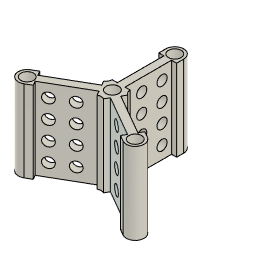
CanSat_MK.2 v2 v7 (Autodesk Fusion 360 archive; units mm, degrees)
design "Module"
Autodesk Fusion 360 part; units mm, degrees
sketch "Sketch1" plane through (0, 0, 0) normal (0, 0, 1) x (1, 0, 0)
  circle A0 centre (0, 0) radius 32
  circle A1 centre (0, 24.5) radius 2.5
  circle A2 centre (-21.2176, -12.25) radius 2.5
  circle A3 centre (21.2176, -12.25) radius 2.5
  circle A4 centre (0, 0) radius 2.5
  line L0 (-3.5, 3.4641) -> (-3.5, 24.5)
  line L1 (3.5, 24.5) -> (3.5, 3.4641)
  line L2 (-1.25, -4.7631) -> (-19.4676, -15.2811)
  line L3 (-22.9676, -9.2189) -> (-4.75, 1.299)
  line L4 (4.75, 1.299) -> (22.9676, -9.2189)
  line L5 (19.4676, -15.2811) -> (1.25, -4.7631)
  arc A5 (-4.75, 1.299) -> (-3.5, 3.4641) centre (-6, 3.4641) ccw
  arc A6 (3.5, 3.4641) -> (4.75, 1.299) centre (6, 3.4641) ccw
  arc A7 (1.25, -4.7631) -> (-1.25, -4.7631) centre (0, -6.9282) ccw
  arc A8 (3.5, 24.5) -> (-3.5, 24.5) centre (0, 24.5) ccw
  arc A9 (19.4676, -15.2811) -> (22.9676, -9.2189) centre (21.2176, -12.25) ccw
  arc A10 (-22.9676, -9.2189) -> (-19.4676, -15.2811) centre (-21.2176, -12.25) ccw
  dimension "d1" = 64
  dimension "d2" = 24.5
  dimension "d3" = 5
  dimension "d5" = 360
  dimension "d6" = 7
  dimension "d8" = 360
  dimension "d10" = 5
  dimension "d15" = 2.5
  dimension "d16" = 2.5
  dimension "d17" = 2.5
  constraint coincident A0.centre A4.centre
  constraint concentric A1 A8
  constraint vertical L0
  constraint vertical L1
  constraint tangent L0 A5
  constraint tangent L3 A5
  constraint tangent L1 A6
  constraint tangent L4 A6
  constraint tangent L5 A7
  constraint tangent L2 A7
  measures "d1" diameter of A0
  measures "d2" distance of A0.centre A1.centre
  measures "d3" diameter of A1
  measures "d6" diameter of A8
  measures "d10" diameter of A4
  measures "d15" radius of A5
  measures "d16" radius of A6
  measures "d17" radius of A7
extrude "Extrude1" add sketch "Sketch1" along normal blind 32 contours L0 L1 L2 L3 L4 L5 A5 A6 A7 A8 A9 A10
sketch "Sketch2" plane through (1.75, -3.0311, 0) normal (0.5, -0.866025, 0) x (0.866025, 0.5, 0)
  line L0 (-24.5, 0) -> (-3.4641, 0)
  line L1 (-3.4641, 0) -> (-3.4641, 32)
  line L2 (-3.4641, 32) -> (-24.5, 32)
  line L3 (-24.5, 32) -> (-24.5, 0)
  line L4 (-24.5, 32) -> (-3.4641, 32)
  line L5 (-3.4641, 32) -> (-3.4641, 0)
  line L6 (-3.4641, 0) -> (-24.5, 0)
  line L7 (-24.5, 0) -> (-24.5, 32)
  circle A0 centre (-18, 27) radius 2
  circle A1 centre (-10, 27) radius 2
  circle A2 centre (-18, 19.6667) radius 2
  circle A3 centre (-10, 19.6667) radius 2
  circle A4 centre (-18, 12.3333) radius 2
  circle A5 centre (-10, 12.3333) radius 2
  circle A6 centre (-18, 5) radius 2
  circle A7 centre (-10, 5) radius 2
  dimension "d20" = 4
  dimension "d23" = 8
  dimension "d24" = -22
  constraint horizontal L4
  constraint vertical L5
  constraint horizontal L6
  constraint vertical L7
  constraint coincident L0.end L1.start
  constraint coincident L2.end L3.start
  measures "d20" diameter of A0
extrude "Extrude2" cut sketch "Sketch2" against normal blind 8 contours A0 | A1 | A2 | A3 | A4 | A5 | A6 | A7
pattern_circular "C-Pattern1" count 3 over 360 about axis through (0, 0, 1.75) along (0, 0, 1) of "Extrude2"
sketch "Sketch3" plane through (1.75, -3.0311, 0) normal (0.5, -0.866025, 0) x (0.866025, 0.5, 0)
  circle A0 centre (-10, 12.3333) radius 2
  circle A1 centre (-10, 27) radius 2
  circle A2 centre (-18, 19.6667) radius 2
  circle A3 centre (-10, 5) radius 2
  circle A4 centre (-18, 12.3333) radius 2
  circle A5 centre (-18, 27) radius 2
  circle A6 centre (-10, 19.6667) radius 2
  circle A7 centre (-18, 5) radius 2
  line L0 (-24.5, 0) -> (-3.4641, 0)
  line L1 (-3.4641, 0) -> (-3.4641, 32)
  line L2 (-3.4641, 32) -> (-24.5, 32)
  line L3 (-24.5, 32) -> (-24.5, 0)
  line L4 (-21.8286, 32) -> (-21.8286, 0)
  constraint coincident L2 L4.start
  constraint coincident L0 L4.end
  constraint perpendicular L0 L4
extrude "Extrude3" cut sketch "Sketch3" against normal blind 2 contours L0 L1 L2 L4
sketch "Sketch5" plane through (-1.75, 3.0311, 0) normal (-0.5, 0.866025, 0) x (-0.866025, -0.5, 0)
  circle A0 centre (10, 12.3333) radius 2
  circle A1 centre (10, 27) radius 2
  circle A2 centre (18, 19.6667) radius 2
  circle A3 centre (10, 5) radius 2
  circle A4 centre (18, 12.3333) radius 2
  circle A5 centre (18, 27) radius 2
  circle A6 centre (10, 19.6667) radius 2
  circle A7 centre (18, 5) radius 2
  line L0 (3.4641, 0) -> (24.5, 0)
  line L1 (24.5, 0) -> (24.5, 32)
  line L2 (24.5, 32) -> (3.4641, 32)
  line L3 (3.4641, 32) -> (3.4641, 0)
  line L4 (24.5, 32) -> (21.829, 32)
  line L5 (21.829, 32) -> (21.829, 0)
  dimension "d31" = 2.671
  constraint coincident L1.end L2.start
  constraint perpendicular L1 L4
  constraint coincident L0 L5.end
  constraint perpendicular L0 L5
  measures "d31" distance of L1.end L4.end
extrude "Extrude4" cut sketch "Sketch5" against normal blind 2 contours L0 L2 L3 L5
sketch "Sketch6" plane through (-3.5, 0, 0) normal (-1, 0, 0) x (0, -1, 0)
  circle A0 centre (-10, 12.3333) radius 2
  circle A1 centre (-10, 27) radius 2
  circle A2 centre (-18, 19.6667) radius 2
  circle A3 centre (-10, 5) radius 2
  circle A4 centre (-18, 12.3333) radius 2
  circle A5 centre (-18, 27) radius 2
  circle A6 centre (-10, 19.6667) radius 2
  circle A7 centre (-18, 5) radius 2
  line L0 (-24.5, 0) -> (-3.4641, 0)
  line L1 (-3.4641, 0) -> (-3.4641, 32)
  line L2 (-3.4641, 32) -> (-24.5, 32)
  line L3 (-24.5, 32) -> (-24.5, 0)
  line L4 (-24.5, 32) -> (-21.739, 32)
  line L5 (-21.739, 32) -> (-21.739, 0)
  dimension "d34" = 2.761
  constraint coincident L2.end L3.start
  constraint perpendicular L3 L4
  constraint coincident L0 L5.end
  constraint perpendicular L0 L5
  measures "d34" distance of L2.end L4.end
extrude "Extrude5" cut sketch "Sketch6" against normal blind 2 contours L0 L1 L2 L5
sketch "Sketch7" plane through (3.5, 0, 0) normal (1, 0, 0) x (0, 1, 0)
  circle A0 centre (10, 12.3333) radius 2
  circle A1 centre (10, 27) radius 2
  circle A2 centre (18, 19.6667) radius 2
  circle A3 centre (10, 5) radius 2
  circle A4 centre (18, 12.3333) radius 2
  circle A5 centre (18, 27) radius 2
  circle A6 centre (10, 19.6667) radius 2
  circle A7 centre (18, 5) radius 2
  line L0 (3.4641, 0) -> (24.5, 0)
  line L1 (24.5, 0) -> (24.5, 32)
  line L2 (24.5, 32) -> (3.4641, 32)
  line L3 (3.4641, 32) -> (3.4641, 0)
  line L4 (24.5, 32) -> (21.739, 32)
  line L5 (21.739, 32) -> (21.739, 0)
  dimension "d37" = 2.761
  constraint coincident L1.end L2.start
  constraint perpendicular L1 L4
  constraint coincident L0 L5.end
  constraint perpendicular L0 L5
  measures "d37" distance of L1.end L4.end
extrude "Extrude6" cut sketch "Sketch7" against normal blind 2 contours L0 L2 L3 L5
sketch "Sketch8" plane through (1.75, 3.0311, 0) normal (0.5, 0.866025, 0) x (-0.866025, 0.5, 0)
  circle A0 centre (-10, 12.3333) radius 2
  circle A1 centre (-10, 27) radius 2
  circle A2 centre (-18, 19.6667) radius 2
  circle A3 centre (-10, 5) radius 2
  circle A4 centre (-18, 12.3333) radius 2
  circle A5 centre (-18, 27) radius 2
  circle A6 centre (-10, 19.6667) radius 2
  circle A7 centre (-18, 5) radius 2
  line L0 (-24.5, 0) -> (-3.4641, 0)
  line L1 (-3.4641, 0) -> (-3.4641, 32)
  line L2 (-3.4641, 32) -> (-24.5, 32)
  line L3 (-24.5, 32) -> (-24.5, 0)
  line L4 (-24.5, 32) -> (-21.739, 32)
  line L5 (-21.739, 32) -> (-21.739, 0)
  dimension "d40" = 2.761
  constraint coincident L2.end L3.start
  constraint perpendicular L3 L4
  constraint coincident L0 L5.end
  constraint perpendicular L0 L5
  measures "d40" distance of L2.end L4.end
extrude "Extrude7" cut sketch "Sketch8" against normal blind 2 contours L0 L1 L2 L5
sketch "Sketch9" plane through (-1.75, -3.0311, 0) normal (-0.5, -0.866025, 0) x (0.866025, -0.5, 0)
  circle A0 centre (10, 12.3333) radius 2
  circle A1 centre (10, 27) radius 2
  circle A2 centre (18, 19.6667) radius 2
  circle A3 centre (10, 5) radius 2
  circle A4 centre (18, 12.3333) radius 2
  circle A5 centre (18, 27) radius 2
  circle A6 centre (10, 19.6667) radius 2
  circle A7 centre (18, 5) radius 2
  line L0 (3.4641, 0) -> (24.5, 0)
  line L1 (24.5, 0) -> (24.5, 32)
  line L2 (24.5, 32) -> (3.4641, 32)
  line L3 (3.4641, 32) -> (3.4641, 0)
  line L4 (24.5, 32) -> (21.739, 32)
  line L5 (21.739, 32) -> (21.739, 0)
  dimension "d43" = 2.761
  constraint coincident L1.end L2.start
  constraint perpendicular L1 L4
  constraint coincident L0 L5.end
  constraint perpendicular L0 L5
  measures "d43" distance of L1.end L4.end
extrude "Extrude8" cut sketch "Sketch9" against normal blind 2 contours L0 L2 L3 L5
sketch "Sketch10" plane through (-0.75, -1.299, 0) normal (-0.5, -0.866025, 0) x (0.866025, -0.5, 0)
  circle A0 centre (10, 27) radius 2
  circle A1 centre (18, 19.6667) radius 2
  circle A2 centre (18, 5) radius 2
  circle A3 centre (10, 12.3333) radius 2
  circle A4 centre (18, 12.3333) radius 2
  circle A5 centre (18, 27) radius 2
  circle A6 centre (10, 19.6667) radius 2
  circle A7 centre (10, 5) radius 2
  line L0 (3.4641, 32) -> (3.4641, 0)
  line L1 (3.4641, 0) -> (21.739, 0)
  line L2 (21.739, 0) -> (21.739, 32)
  line L3 (21.739, 32) -> (3.4641, 32)
